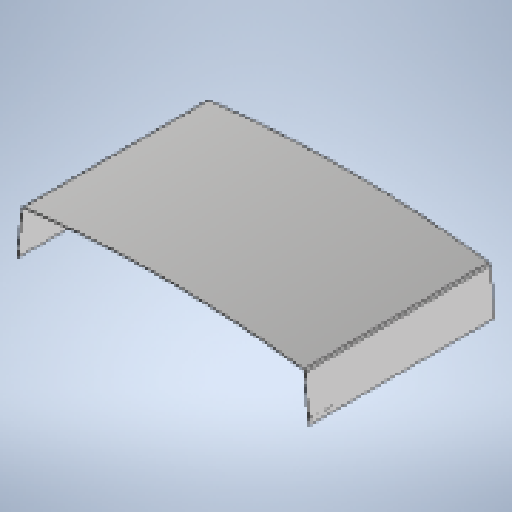
# Autodesk Inventor part: MSC 201 sheet back basic
Saved by Autodesk Inventor 2025 (Build 290162010, 162A)
## iProperties
Created: 2024-04-18
Part Number: MSC 201 sheet back basic
Material: Stainless Steel AISI 304
Document SubType Name: Sheet Metal
Designer: admin
Density: 8 g/cm^3
Sheet Metal Rule: AISI304 3mm Die 32
Sheet Metal Width: 980,000 mm
Sheet Metal Length: 1980,030 mm
Sheet Metal Area: 1940429,794 mm^2
Appearance: Default
Stock Number: МОО 201 лист спина базовый
Mass: 46582.9 g
Surface Area: 38996.7 cm^2
Volume: 5822.86 cm^3
Flat Pattern Width: 98 cm
Flat Pattern Length: 198.003 cm
Flat Pattern Area: 19404.3 cm^2
Author: admin
Autodesk Inventor part; units mm, degrees
ref_plane "YZ Plane" through (0, 0, 0) normal (1, 0, 0) x (0, 1, 0)
ref_plane "XZ Plane" through (0, 0, 0) normal (0, 1, 0) x (-1, 0, 0)
ref_plane "XY Plane" through (0, 0, 0) normal (0, 0, 1) x (1, 0, 0)
sketch "Sketch1" plane through (0, 0, 0) normal (0, 0, 1) x (1, 0, 0)
  line L0 (-750, 0) -> (750, 0) construction
  line L1 (750, 0) -> (750, -2700) construction
  line L2 (750, -2700) -> (-750, -2700) construction
  line L3 (-750, -2700) -> (-750, 0) construction
  line L4 (800, 50) -> (-800, 50) construction
  line L5 (-800, 50) -> (-800, -2750) construction
  line L6 (-800, -2750) -> (800, -2750) construction
  line L7 (800, -2750) -> (800, 50) construction
  line L8 (-850, 100) -> (850, 100) construction
  line L9 (850, 100) -> (850, -2800) construction
  line L10 (850, -2800) -> (-850, -2800) construction
  line L11 (-850, -2800) -> (-850, 100) construction
  arc A0 (750, 0) -> (742.111681, 1.050817) centre (0, -5600) ccw construction
  line L12 (-750, -2100) -> (750, -2100) construction
  line L13 (115.485997, -2697.8227) -> (750, -2100) construction
  arc A1 (750, -2100) -> (750, 0) centre (-10250, -1050) ccw construction
  arc A2 (110, -2700) -> (115.485997, -2697.8227) centre (110, -2692) ccw construction
  arc A3 (742.111681, 1.050817) -> (0, 50) centre (0, -5600) ccw
  line L14 (0, 100) -> (0, 50) construction
  line L15 (0, -2700) -> (0, -2697) construction
  line L16 (0, 47) -> (0, 0) construction
  line L17 (0, 50) -> (0, 47) construction
  line L18 (750.763103, -8.025362) -> (770.411716, -241.9)
  arc A4 (750.763103, -8.025362) -> (742.111681, 1.050817) centre (740.798209, -8.862547) ccw
  point P0 (0, -2750)
  dimension "d54" = 1500
  dimension "d55" = 2700
  dimension "d58" = 2100
  dimension "d83" = 8
  dimension "d113" = 50
  dimension "d114" = 50
  dimension "d115" = 3
  dimension "d121" = 10
  dimension "d122" = 241.9
  dimension "d124" = 94.8023
  measures "d54" distance of L0.start L0.end
  measures "d55" distance of L0.end L1.end
  measures "d58" distance between parallel lines of L12 L0
  measures "d83" radius of A2
  measures "d113" distance between parallel lines of L4 L8
  measures "d114" distance between parallel lines of L0 L4
  measures "d115" distance of L14.end L16.start
  measures "d121" radius of A4
  measures "d122" vertical distance of L18.end L0.end
  measures "d124" angle of L0 L18
contour flange "Contour Flange2" sketch "Sketch1" thickness 3 bend radius 5 width 980 along (0, 0, 1) mid plane no both sides no wall seen from (760.58741, -124.962681, 0) lies toward (-0.9964894, -0.0837185, 0) curves L18 A4 A3
bend "Bend2"
corner "Corner2"
mirror "Mirror2" about plane through (0, 0, 0) normal (1, 0, 0) of "Contour Flange2"
sketch "Sketch2" plane through (747.773635, -8.276518, 0) normal (-0.9964894, -0.0837185, 0) x (0, 0, 1)
  line L0 (963.847804, -212.844904) -> (852.423188, -212.844904) construction
  line L1 (852.423188, -212.844904) -> (852.423188, -183.740468) construction
  line L2 (852.423188, -183.740468) -> (963.847804, -183.740468) construction
  line L3 (963.847804, -183.740468) -> (963.847804, -212.844904) construction
  point P0 (0, 70.849954)
  constraints: 2 other
mark "Mark1"
equation "\"d36\" = Thickness"
equation "\"d37\" = BendReliefWidth"
equation "\"d38\" = BendReliefDepth"
equation "\"d39\" = MinimumRemnant"
equation "\"d40\" = TransitionRadius"
equation "\"d42\" = BendRadius"
equation "\"d44\" = CornerReliefSize"
equation "\"d45\" = GapSize"
equation "\"d46\" = JacobiRadiusSize"
equation "\"BendReliefWidth\" = Thickness"
equation "\"BendReliefDepth\" = 0.5 * Thickness"
equation "\"CornerReliefSize\" = 4 * Thickness"
equation "\"MinimumRemnant\" = 2 * Thickness"
equation "\"GapSize\" = Thickness"
equation "\"Thickness\" = 3"
equation "\"TransitionRadius\" = 5"
equation "\"BendRadius\" = 5"
equation "\"JacobiRadiusSize\" = 5"
body "Solid3"
